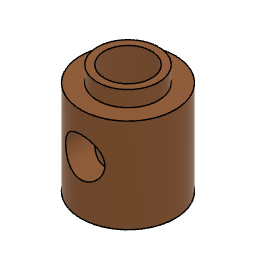
pulse transfer insulator v2 (Autodesk Fusion 360 design; units mm, degrees)
Autodesk Fusion 360 part; units mm, degrees
cylinder "CylinderPrimitive1" add diameter 6 height 6 placed x (1, 0, 0) y (0, 0, -1) z (0, 1, 0) at (0, 0, 0)
cylinder "CylinderPrimitive2" add diameter 3.9 height 1 placed x (1, 0, 0) y (0, 0, -1) z (0, 1, 0) at (0, 6, 0)
hole "Hole1" at (0, 7, 0) direction (0, -1, 0) diameter 3 end through all
hole "Hole2" at (0, 3.3861, 3) direction (0, 0, -1) diameter 2.5 depth 7 tip angle 118
